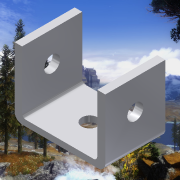
# Autodesk Inventor part: C19_TK_ClimberingSupportBracket
Saved by Autodesk Inventor 2015 SP1 (Build 190203100, 203)
## iProperties
Created: 2015-01-17
Part Number: C19_TK_ClimberingSupportBracket
Material: Aluminum 6061
Document SubType Name: Modeling
Designer: Administrator
Density: 2.7 g/cm^3
Appearance: Aluminum - Flat
Mass: 17.3242 g
Surface Area: 51.2712 cm^2
Volume: 6.41638 cm^3
Author: Administrator
Autodesk Inventor part; units mm, degrees
ref_plane "YZ Plane" through (0, 0, 0) normal (1, 0, 0) x (0, 1, 0)
ref_plane "XZ Plane" through (0, 0, 0) normal (0, 1, 0) x (-1, 0, 0)
ref_plane "XY Plane" through (0, 0, 0) normal (0, 0, 1) x (1, 0, 0)
sketch "Sketch1" plane through (0, 0, 0) normal (0, 0, 1) x (1, 0, 0)
  line L0 (-15.9912, -11.7475) -> (15.7588, -11.7475)
  line L1 (15.7588, -11.7475) -> (15.7588, 14.2875)
  line L2 (-15.9912, 14.2875) -> (-15.9912, -11.7475)
  line L3 (-15.9912, -11.7475) -> (15.7588, 11.5768) construction
  line L4 (15.7588, -11.7475) -> (-15.9912, 11.9207) construction
  line L5 (19.1662, -14.2875) -> (-19.1662, -14.2875)
  line L6 (-19.1662, -14.2875) -> (-19.1662, 14.2875)
  line L7 (19.1662, 14.2875) -> (19.1662, -14.2875)
  line L8 (19.1662, -14.2875) -> (-19.1662, 14.2875) construction
  line L9 (-19.1662, -14.2875) -> (19.1662, 14.2875) construction
  line L10 (-19.1662, 14.2875) -> (-15.9912, 14.2875)
  line L11 (15.7588, 14.2875) -> (19.1662, 14.2875)
  point P0 (0, 0)
  dimension "d2" = 3.175
  dimension "d3" = 28.575
  dimension "d4" = 31.75
  dimension "d5" = 2.54
  constraints: 24 end point, 5 parallel, 5 point on line, 2 horizontal, 2 midpoint, 2 perpendicular
  measures "d2" distance between parallel lines of L2 L6
  measures "d3" distance between parallel lines of L10 L5
  measures "d4" distance between parallel lines of L1 L2
  measures "d5" distance between parallel lines of L5 L0
extrude "Extrusion1" add sketch "Sketch1" along normal mid plane 25.4
sketch "Sketch2" plane through (19.1662, 14.2875, 12.7) normal (1, 0, 0) x (0, 0, -1)
  line L0 (0, 0) -> (25.4, 0) projected
  point P0 (12.7, -14.2875)
  point P1 (12.7, -12.7)
  dimension "d9" = 12.7
  measures "d9" distance from line of L0 point (12.7, -12.7)
hole "Hole1" at (19.1662, 1.5875, 0) direction (-1, 0, 0) diameter 6.7564 end through all clearance for "Flat Head Machine Screw (82)" size "1/4" standard "Ansi Unified Screw Threads"
sketch "Sketch3" plane through (-15.9912, -11.7475, 12.7) normal (0, 1, 0) x (1, 0, 0)
  line L0 (0, 25.4) -> (0, 0) projected
  line L1 (0, 25.4) -> (31.75, 25.4) projected
  point P0 (15.875, 12.7)
  point P1 (15.875, 12.7)
  dimension "d26" = 12.7
  dimension "d27" = 15.875
  constraints: 1 coincident
  measures "d26" distance from line of L1 point (15.875, 12.7)
  measures "d27" distance from line of L0 point (15.875, 12.7)
hole "Hole2" at (-0.1162, -11.7475, 0) direction (0, -1, 0) diameter 6.7564 end through all clearance for "Flat Head Machine Screw (82)" size "1/4" standard "Ansi Unified Screw Threads"
fillet "Fillet2" radius 3.175 2 edges at (-19.1662, -14.2875, 0) (19.1662, -14.2875, 0)
fillet "Fillet3" radius 1.5875 2 edges at (-15.9912, -11.7475, 0) (15.7588, -11.7475, 0)
sketch "Sketch4" plane through (-19.1662, 14.2875, -12.7) normal (-1, 0, 0) x (0, 0, 1)
  circle A0 centre (12.7, -12.7) radius 3.3782 projected
  circle A1 centre (12.7, -12.7) radius 728.218
  line L0 (723.9, -1.1049) -> (723.9, 7.4549) projected
  circle A2 centre (653.833, 332.6257) radius 3.5687 projected
  point P0 (12.7, -14.2875)
  point P1 (723.9, 143.812)
  constraints: 2 point on circle, 1 centre point, 1 coincident, 1 point on line
body "Solid1"
